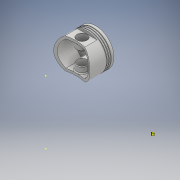
# Autodesk Inventor part: Part3
Saved by Autodesk Inventor 2019 (Build 230136000, 136)
## iProperties
Created: 2017-10-05
Part Number: Part3
Material: Generic
Document SubType Name: Modeling
Designer: Usuario
Density: 1 g/cm^3
Appearance: Default
Author: Usuario
Autodesk Inventor part; units mm, degrees
ref_plane "YZ Plane" through (0, 0, 0) normal (1, 0, 0) x (0, 1, 0)
ref_plane "XZ Plane" through (0, 0, 0) normal (0, 1, 0) x (-1, 0, 0)
ref_plane "XY Plane" through (0, 0, 0) normal (0, 0, 1) x (1, 0, 0)
sketch "Sketch1" plane through (0, 0, 0) normal (0, 1, 0) x (-1, 0, 0)
  circle A0 centre (0, 0) radius 40
  dimension "d0" = 80
  constraints: 1 centre point, 1 coincident
  measures "d0" diameter of A0
extrude "Extrusion1" add sketch "Sketch1" along normal blind 53
sketch "Sketch2" plane through (0, 0, 0) normal (1, 0, 0) x (0, 1, 0)
  line L0 (0, 40) -> (53, 40) projected
  line L1 (53, 40) -> (53, -40) projected
  line L2 (53, -40) -> (0, -40) projected
  line L3 (0, -40) -> (0, 40) projected
  line L4 (0, 40) -> (34, 40)
  line L5 (34, 40) -> (34, 33.5)
  line L6 (34, 33.5) -> (0, 33.5)
  line L7 (0, 33.5) -> (0, 40)
  point P0 (0, 0)
  dimension "d3" = 6.5
  dimension "d4" = 19
  constraints: 8 end point, 2 parallel, 1 horizontal, 1 perpendicular
  measures "d3" distance between parallel lines of L0 L6
  measures "d4" distance between parallel lines of L1 L5
extrude "Extrusion2" cut sketch "Sketch2" along normal mid plane 53 contours L0 L5 L6 L3
mirror "Mirror1" about plane through (0, 0, 0) normal (0, 0, 1) of "Extrusion2"
sketch "Sketch3" plane through (0, 53, 0) normal (0, 1, 0) x (1, 0, 0)
  circle A0 centre (0, 0) radius 34
  dimension "d7" = 68
  constraints: 1 centre point, 1 coincident
  measures "d7" diameter of A0
extrude "Extrusion3" cut sketch "Sketch3" against normal blind 1
sketch "Sketch4" plane through (0, 0, 0) normal (0, 0, 1) x (1, 0, 0)
  line L0 (40, 0) -> (40, 53) projected
  line L1 (40, 47) -> (38, 47)
  line L2 (38, 47) -> (38, 45.5)
  line L3 (38, 45.5) -> (40, 45.5)
  line L4 (40, 42.5) -> (38, 42.5)
  line L5 (38, 42.5) -> (38, 41)
  line L6 (38, 41) -> (40, 41)
  line L7 (40, 38) -> (38, 38)
  line L8 (38, 38) -> (38, 36.5)
  line L9 (38, 36.5) -> (40, 36.5)
  line L10 (40, 53) -> (-40, 53) projected
  line L11 (0, -10.6) -> (0, 63.6) projected
  point P0 (0, 0)
  dimension "d10" = 3
  dimension "d11" = 2
  dimension "d12" = 1.5
  dimension "d13" = 1.5
  dimension "d14" = 1.5
  dimension "d15" = 3
  dimension "d16" = 6
  constraints: 18 end point, 10 point on line, 5 perpendicular, 2 parallel
  measures "d10" distance between parallel lines of L4 L3
  measures "d11" distance between parallel lines of L0 L2
  measures "d12" distance of L1.end L2.end
  measures "d13" distance of L4.end L5.end
  measures "d14" distance of L7.end L8.end
  measures "d15" distance between parallel lines of L6 L7
  measures "d16" distance between parallel lines of L10 L1
revolve "Revolution1" cut sketch "Sketch4" angle 360 about axis through (0, -10, 0) along (0, 1, 0)
sketch "Sketch5" plane through (0, 0, 0) normal (0, 0, 1) x (1, 0, 0)
  point P0 (0, 0)
sketch "Sketch6" plane through (0, 0, 0) normal (0, -1, 0) x (1, 0, 0)
  line L0 (21.8575, -33.5) -> (-21.8575, -33.5) projected
  arc A0 (-21.8575, 33.5) -> (-21.8575, -33.5) centre (0, 0) ccw projected
  line L1 (-21.8575, 33.5) -> (21.8575, 33.5) projected
  arc A1 (21.8575, -33.5) -> (21.8575, 33.5) centre (0, 0) ccw projected
  line L2 (20.1556, 28) -> (-20.1556, 28)
  arc A2 (-20.1556, 28) -> (-20.1556, -28) centre (0, 0) ccw
  line L3 (-20.1556, -28) -> (20.1556, -28)
  arc A3 (20.1556, -28) -> (20.1556, 28) centre (0, 0) ccw
  dimension "d18" = 5.5
  constraints: 4 end point, 4 point on circle, 2 centre point, 3 other
  measures "d18" distance between parallel lines of L1 L2
extrude "Extrusion4" cut sketch "Sketch6" against normal blind 43 contours A3 L3 A2 L2
sketch "Sketch7" plane through (21.8575, 0, -33.5) normal (0, 0, -1) x (-1, 0, 0)
  line L0 (61.8575, 53) -> (-18.1425, 53) projected
  line L1 (0, 0) -> (0, 34) projected
  line L2 (43.715, 0) -> (0, 0) projected
  line L3 (43.715, 34) -> (43.715, 0) projected
  line L4 (43.715, 34) -> (0, 34) projected
  circle A0 centre (21.8575, 22.5) radius 9.5
  point P0 (21.8575, 0)
  point P1 (21.8575, 53)
  dimension "d21" = 30.5
  dimension "d22" = 19
  dimension "d23" = 43.715
  constraints: 1 centre point, 1 coincident, 1 midpoint, 1 vertical alignment
  measures "d21" distance from line of point (21.857, 22.5) L0
  measures "d22" diameter of A0
  measures "d23" distance of L2.start L1.start
extrude "Extrusion5" cut sketch "Sketch7" against normal through all contours A0
sketch "Sketch8" plane through (21.8575, 0, -33.5) normal (0, 0, -1) x (-1, 0, 0)
  line L0 (-18.1425, 0) -> (0, 0) projected
  line L1 (43.715, 0) -> (61.8575, 0) projected
  line L2 (43.715, 0) -> (0, 0) projected
  line L3 (21.8575, 0) -> (21.8575, 19)
  arc A0 (61.8575, 0) -> (-18.1425, 0) centre (21.8575, -79.4605) ccw
  line L4 (-18.1425, 0) -> (61.8575, 0)
  point P0 (21.8575, 9.5)
  dimension "d27" = 9.5
  constraints: 4 end point, 3 point on circle, 1 centre point, 1 midpoint, 1 vertical
  measures "d27" distance from line of point (21.857, 9.5) L2
extrude "Extrusion6" cut sketch "Sketch8" against normal up to next
sketch "Sketch9" plane through (20.1556, 43, 28) normal (0, 0, -1) x (-1, 0, 0)
  circle A0 centre (20.1556, -20.5) radius 9.5 projected
  line L0 (0.8683, 10) -> (0.8683, 9) projected
  line L1 (0.8683, 9) -> (39.4429, 9) projected
  line L2 (39.4429, 9) -> (39.4429, 10) projected
  line L3 (39.4429, 10) -> (48.7214, 10) projected
  line L4 (48.7214, 10) -> (48.7214, 4) projected
  line L5 (48.7214, 4) -> (45.8461, 4) projected
  line L6 (45.8461, 4) -> (45.8461, 2.5) projected
  line L7 (45.8461, 2.5) -> (48.7214, 2.5) projected
  line L8 (48.7214, 2.5) -> (48.7214, -0.5) projected
  line L9 (48.7214, -0.5) -> (45.8461, -0.5) projected
  line L10 (45.8461, -0.5) -> (45.8461, -2) projected
  line L11 (45.8461, -2) -> (48.7214, -2) projected
  line L12 (48.7214, -2) -> (48.7214, -5) projected
  line L13 (48.7214, -5) -> (45.8461, -5) projected
  line L14 (45.8461, -5) -> (45.8461, -6.5) projected
  line L15 (45.8461, -6.5) -> (48.7214, -6.5) projected
  line L16 (48.7214, -6.5) -> (48.7214, -38.211) projected
  arc A1 (48.7214, -38.211) -> (40.3113, -35.8134) centre (20.1556, -122.4605) ccw projected
  arc A2 (40.3113, -35.8134) -> (0, -35.8134) centre (20.1556, -122.4605) ccw projected
  arc A3 (0, -35.8134) -> (-8.4101, -38.211) centre (20.1556, -122.4605) ccw projected
  line L17 (-8.4101, -38.211) -> (-8.4101, -6.5) projected
  line L18 (-8.4101, -6.5) -> (-5.5348, -6.5) projected
  line L19 (-5.5348, -6.5) -> (-5.5348, -5) projected
  line L20 (-5.5348, -5) -> (-8.4101, -5) projected
  line L21 (-8.4101, -5) -> (-8.4101, -2) projected
  line L22 (-8.4101, -2) -> (-5.5348, -2) projected
  line L23 (-5.5348, -2) -> (-5.5348, -0.5) projected
  line L24 (-5.5348, -0.5) -> (-8.4101, -0.5) projected
  line L25 (-8.4101, -0.5) -> (-8.4101, 2.5) projected
  line L26 (-8.4101, 2.5) -> (-5.5348, 2.5) projected
  line L27 (-5.5348, 2.5) -> (-5.5348, 4) projected
  line L28 (-5.5348, 4) -> (-8.4101, 4) projected
  line L29 (-8.4101, 4) -> (-8.4101, 10) projected
  line L30 (-8.4101, 10) -> (0.8683, 10) projected
  line L31 (40.3113, -35.8134) -> (40.3113, 0) projected
  line L32 (40.3113, 0) -> (0, 0) projected
  line L33 (0, 0) -> (0, -35.8134) projected
  circle A4 centre (20.1556, -20.5) radius 9.5
  arc A5 (8.6556, -20.5) -> (31.6556, -20.5) centre (20.1556, -20.5) ccw
  line L34 (8.6556, -20.5) -> (8.6556, 0)
  line L35 (31.6556, -20.5) -> (31.6556, 0)
  line L36 (8.6556, 0) -> (31.6556, 0)
  point P0 (20.1556, -43)
  dimension "d30" = 19
  dimension "d31" = 23
  constraints: 6 end point, 2 centre point, 2 coincident, 2 perpendicular, 2 point on circle, 2 point on line, 2 tangent, 1 collinear
  measures "d30" diameter of A4
  measures "d31" diameter of A5
extrude "Extrusion7" add sketch "Sketch9" along normal blind 14 contours L32 L35 A5 L34
mirror "Mirror2" about plane through (0, 0, 0) normal (0, 0, 1) of "Extrusion7"
sketch "Sketch10" plane through (21.8575, 34, -33.5) normal (0, 0, -1) x (-1, 0, 0)
  point P0 (21.8575, -34)
sketch "Sketch11" plane through (21.8575, 34, -33.5) normal (0, 0, -1) x (-1, 0, 0)
  circle A0 centre (21.8575, -11.5) radius 9.5 projected
  line L0 (27.667, 18) -> (27.667, 19) projected
  line L1 (27.667, 19) -> (43.715, 19) projected
  line L2 (43.715, 19) -> (43.715, 13) projected
  line L3 (43.715, 13) -> (39.7949, 13) projected
  line L4 (39.7949, 13) -> (39.7949, 11.5) projected
  line L5 (39.7949, 11.5) -> (43.715, 11.5) projected
  line L6 (43.715, 11.5) -> (43.715, 8.5) projected
  line L7 (43.715, 8.5) -> (39.7949, 8.5) projected
  line L8 (39.7949, 8.5) -> (39.7949, 7) projected
  line L9 (39.7949, 7) -> (43.715, 7) projected
  line L10 (43.715, 7) -> (43.715, 4) projected
  line L11 (43.715, 4) -> (39.7949, 4) projected
  line L12 (39.7949, 4) -> (39.7949, 2.5) projected
  line L13 (39.7949, 2.5) -> (43.715, 2.5) projected
  line L14 (43.715, 2.5) -> (43.715, 0) projected
  line L15 (43.715, 0) -> (43.715, -27.227) projected
  arc A1 (43.715, -27.227) -> (0, -27.227) centre (21.8575, -113.4605) ccw projected
  line L16 (0, -27.227) -> (0, 0) projected
  line L17 (43.715, 0) -> (0, 0) projected
  line L18 (16.048, 18) -> (27.667, 18) projected
  line L19 (16.048, 19) -> (16.048, 18) projected
  line L20 (0, 19) -> (16.048, 19) projected
  line L21 (0, 13) -> (0, 19) projected
  line L22 (3.9201, 13) -> (0, 13) projected
  line L23 (3.9201, 11.5) -> (3.9201, 13) projected
  line L24 (0, 11.5) -> (3.9201, 11.5) projected
  line L25 (0, 8.5) -> (0, 11.5) projected
  line L26 (3.9201, 8.5) -> (0, 8.5) projected
  line L27 (3.9201, 7) -> (3.9201, 8.5) projected
  line L28 (0, 7) -> (3.9201, 7) projected
  line L29 (0, 4) -> (0, 7) projected
  line L30 (3.9201, 4) -> (0, 4) projected
  line L31 (3.9201, 2.5) -> (3.9201, 4) projected
  line L32 (0, 2.5) -> (3.9201, 2.5) projected
  line L33 (0, 0) -> (0, 2.5) projected
  circle A2 centre (21.8575, -11.5) radius 9.5
  circle A3 centre (21.8575, -11.5) radius 10.25
  point P0 (21.8575, -34)
  dimension "d34" = 19
  dimension "d35" = 20.5
  constraints: 2 centre point, 2 coincident
  measures "d34" diameter of A2
  measures "d35" diameter of A3
extrude "Extrusion8" cut sketch "Sketch11" against normal blind 3 contours A3
extrude "Extrusion9" add sketch "Sketch11" against normal blind 2 contours A3
extrude "Extrusion10" cut sketch "Sketch11" against normal blind 1 contours A3
mirror "Mirror4" about plane through (0, 0, 0) normal (0, 0, 1) of "Extrusion9", "Extrusion8", "Extrusion10"
chamfer "Chamfer1" distance 1 angle 45 2 edges at (10.25, 22.5, -33.5) (10.25, 22.5, 33.5)
fillet "Fillet1" radius 2 3 edges at (0, 11, -14) (-11.5, 32.75, -14) (11.5, 32.75, -14)
fillet "Fillet2" radius 2 3 edges at (0, 11, 14) (11.5, 32.75, 14) (-11.5, 32.75, 14)
fillet "Fillet3" radius 2 6 edges at (0, 11, 28) (11.5, 32.75, 28) (-11.5, 32.75, 28) (-11.5, 32.75, -28) (11.5, 32.75, -28) (0, 11, -28)
scale "Scale1" factors (0.24, 0.24, 0.24) then translate (0, 13.87, 0) bodies 1
sketch "Sketch12" plane through (5.2458, 22.03, -8.04) normal (0, 0, -1) x (-1, 0, 0)
  circle A0 centre (5.2458, -2.76) radius 2.7 projected
  circle A1 centre (5.2458, -2.76) radius 2.52
  point P0 (5.2458, -22.03)
  dimension "d51" = 5.04
  constraints: 1 centre point, 1 coincident
  measures "d51" diameter of A1
extrude "Extrusion11" cut sketch "Sketch12" against normal blind 24 contours A1
body "Solid1"
